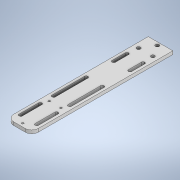
# Autodesk Inventor part: Adapter_Handgelenk_HallsensorHalter
Saved by Autodesk Inventor 2022.2 (Build 262287010, 287A)
## iProperties
Created: 2024-02-12
Part Number: Adapter_Handgelenk_HallsensorHalter
Material: Generisch
Document SubType Name: Modeling
Designer: ppovolni
Density: 1 g/cm^3
Appearance: Vorgabe
Author: ppovolni
Autodesk Inventor part; units mm, degrees
ref_plane "Arbeitsebene1" through (19.8074, 22.7962, -37.1968) normal (0, 1, 0) x (-1, 0, 0)
sketch "Skizze1" plane through (19.8074, 22.7962, -37.1968) normal (0, 1, 0) x (-1, 0, 0)
  circle A0 centre (8, 25) radius 2.8 projected
  circle A1 centre (30, 25) radius 2.8 projected
  circle A2 centre (19, 7) radius 2.8 projected
  spline S0 degree 3 poles (1.3145, 2) (1.0175, 2) (0.7205, 1.9713) (0.2844, 1.885) (0.1411, 1.8492) (0, 1.8064) knots 2.611891 2.611891 2.611891 2.611891 2.701 2.701 2.745234 2.745234 2.745234 2.745234 projected
  line L0 (36.6855, 2) -> (1.3145, 2) projected
  spline S1 degree 3 poles (38, 1.8064) (37.5746, 1.9355) (37.13, 2) (36.6855, 2) knots 0.725365 0.725365 0.725365 0.725365 0.858708 0.858708 0.858708 0.858708 projected
  line L1 (38, 1.8064) -> (38, 28) projected
  spline S2 degree 3 poles (35.7631, 30) (36.052, 30) (36.3933, 29.9384) (36.9135, 29.7364) (37.1885, 29.5671) (37.5676, 29.2109) (37.7437, 28.9664) (37.9403, 28.5182) (38, 28.2384) (38, 28) knots 0.951911 0.951911 0.951911 0.951911 1.038602 1.038602 1.119337 1.119337 1.19466 1.19466 1.266177 1.266177 1.266177 1.266177 projected
  line L2 (2.2369, 30) -> (35.7631, 30) projected
  spline S3 degree 3 poles (0, 28) (0, 28.2384) (0.0597, 28.5182) (0.2563, 28.9664) (0.4324, 29.2109) (0.8115, 29.5671) (1.0865, 29.7364) (1.6067, 29.9384) (1.948, 30) (2.2369, 30) knots 1.266177 1.266177 1.266177 1.266177 1.337694 1.337694 1.413017 1.413017 1.493752 1.493752 1.580443 1.580443 1.580443 1.580443 projected
  line L3 (0, 1.8064) -> (0, 28) projected
  point P0 (19.8074, 37.1968)
ref_plane "Arbeitsebene2" through (19.8074, 22.7962, -37.1968) normal (0, 1, 0) x (-1, 0, 0)
sketch "Skizze2" plane through (19.8074, 22.7962, -37.1968) normal (0, 1, 0) x (-1, 0, 0)
  line L0 (38, 220) -> (0, 220)
  line L1 (0, 220) -> (0, 2)
  line L2 (0, 2) -> (38, 2)
  line L3 (38, 2) -> (38, 220)
  line L4 (38, 1.8064) -> (38, 28) construction
  line L5 (36.6855, 2) -> (1.3145, 2) construction
  line L6 (0, 1.8064) -> (0, 28) construction
  circle A0 centre (8, 25) radius 2.8 construction
  circle A1 centre (19, 7) radius 2.8 construction
  circle A2 centre (19, 7) radius 2.8 construction
  circle A3 centre (30, 25) radius 2.8 construction
  line L7 (24, 205) -> (14, 205) construction
  line L8 (14, 205) -> (14, 185) construction
  line L9 (14, 185) -> (24, 185) construction
  line L10 (24, 185) -> (24, 205) construction
  circle A4 centre (24, 205) radius 1 construction
  circle A5 centre (14, 205) radius 1 construction
  circle A6 centre (24, 185) radius 1 construction
  circle A7 centre (14, 185) radius 1 construction
  line L11 (28, 215) -> (10, 215) construction
  line L12 (10, 215) -> (10, 165) construction
  line L13 (10, 165) -> (28, 165) construction
  line L14 (28, 165) -> (28, 215) construction
  circle A8 centre (28, 165) radius 1.55
  circle A9 centre (10, 165) radius 1.55
  circle A10 centre (19, 215) radius 1.55
  line L15 (5.3985, -5) -> (32.6015, -5) construction
  circle A11 centre (30, 25) radius 2.8 projected
  circle A12 centre (19, 7) radius 2.8 projected
  circle A13 centre (8, 25) radius 2.8 projected
  point P0 (19.8074, 37.1968)
  point P1 (19, 205)
  point P2 (19, 220)
  dimension "d0" = 10
  dimension "d1" = 20
  dimension "d2" = 2
  dimension "d3" = 10
  dimension "d4" = 18
  dimension "d5" = 50
  dimension "d6" = 3.1
  dimension "d8" = 220
  dimension "d9" = 5
  constraints: 24 end point, 7 centre point, 7 coincident, 6 parallel, 5 equal radius, 3 collinear, 3 horizontal, 3 midpoint, 3 perpendicular, 2 vertical alignment
  measures "d0" distance of L7.start L7.end
  measures "d1" distance of L9.end L7.start
  measures "d2" diameter of A5
  measures "d3" distance between parallel lines of L11 L7
  measures "d4" distance of L11.start L11.end
  measures "d5" distance of L13.end L11.start
  measures "d6" diameter of A8
  measures "d8" distance between parallel lines of L11 L15
  measures "d9" distance between parallel lines of L0 L11
extrude "Extrusion1" add sketch "Skizze2" along normal blind 5
sketch "Skizze3" plane through (19.8074, 22.7962, -37.1968) normal (0, -1, 0) x (1, 0, 0)
  line L0 (-15, 30) -> (-23, 30)
  line L1 (-23, 30) -> (-23, 210)
  line L2 (-23, 210) -> (-15, 210)
  line L3 (-15, 210) -> (-15, 30)
  line L4 (-38, 220) -> (0, 220) construction
  line L5 (-29.247, 30) -> (-8.753, 30) construction
  point P0 (-19.8074, 37.1968)
  point P1 (-19, 210)
  point P2 (-19, 220)
  point P3 (-19, 30)
  dimension "d12" = 0
  dimension "d13" = 8
  dimension "d14" = 10
  constraints: 8 end point, 3 midpoint, 2 parallel, 1 horizontal, 1 perpendicular, 1 vertical alignment
  measures "d12" distance from line of point (-19, 30) L5
  measures "d13" distance between parallel lines of L1 L3
  measures "d14" distance from line of L4 point (-19, 210)
ref_plane "Arbeitsebene3" through (-12.7983, 15.7405, -42.1968) normal (0, -1, 0) x (1, 0, 0)
extrude "Extrusion2" add sketch "Skizze3" along normal blind 10
fillet "Rundung1" radius 2 3 edges at (-3.1926, 22.7962, 82.8032) (0.8074, 22.7962, 172.8032) (4.8074, 22.7962, 82.8032)
fillet "Rundung2" radius 10 2 edges at (-18.1926, 25.2962, 182.8032) (19.8074, 25.2962, 182.8032)
fillet "Rundung3" radius 2 4 edges at (-3.1926, 12.7962, 82.8032) (0.8074, 12.7962, 172.8032) (4.8074, 12.7962, 82.8032) (0.8074, 12.7962, -7.1968)
sketch "Skizze4" plane through (19.8074, 22.7962, -37.1968) normal (0, 1, 0) x (1, 0, 0)
  line L0 (-28, -102) -> (-28, -62) construction
  line L1 (-38, -2) -> (-38, -220) construction
  line L2 (0, -2) -> (-38, -2) construction
  line L3 (-28, -71.0877) -> (-28, -66.6042)
  line L4 (-28, -66.6042) -> (-28.9936, -66.6042)
  spline S0 degree 2 poles (-28.9936, -66.6042) (-29.4484, -67.1727) (-30.2492, -68.0822) (-30.61, -68.4233) knots 0 0 0 1 2 2 2
  spline S1 degree 2 poles (-30.61, -68.4233) (-31.0797, -68.8731) (-31.7964, -69.2735) (-32.1721, -69.2735) knots 0 0 0 1 2 2 2
  spline S2 degree 2 poles (-32.1721, -69.2735) (-32.5972, -69.2735) (-33.052, -68.7644) (-33.052, -68.3096) knots 0 0 0 1 2 2 2
  spline S3 degree 2 poles (-33.052, -68.3096) (-33.052, -68.0773) (-32.9383, -67.662) (-32.8494, -67.4495) knots 0 0 0 1 2 2 2
  spline S4 degree 2 poles (-32.8494, -67.4495) (-32.7554, -67.2419) (-32.5577, -66.9453) (-32.5083, -66.8711) knots 0 0 0 1 2 2 2
  line L5 (-32.5083, -66.8711) -> (-32.5083, -66.7525)
  line L6 (-32.5083, -66.7525) -> (-33.838, -66.7525)
  spline S5 degree 2 poles (-33.838, -66.7525) (-33.9616, -67.0095) (-34.2186, -68.1069) (-34.2186, -68.6161) knots 0 0 0 1 2 2 2
  spline S6 degree 2 poles (-34.2186, -68.6161) (-34.2186, -69.7036) (-33.2498, -70.8208) (-32.3748, -70.8208) knots 0 0 0 1 2 2 2
  spline S7 degree 2 poles (-32.3748, -70.8208) (-31.836, -70.8208) (-30.7979, -70.3116) (-30.2047, -69.7234) knots 0 0 0 1 2 2 2
  spline S8 degree 2 poles (-30.2047, -69.7234) (-29.8389, -69.3526) (-29.2704, -68.6556) (-29.1518, -68.5024) knots 0 0 0 1 2 2 2
  line L7 (-29.1518, -68.5024) -> (-29.1518, -71.0877)
  line L8 (-29.1518, -71.0877) -> (-28, -71.0877)
  line L9 (-28, -76.4314) -> (-28, -71.9479)
  line L10 (-28, -71.9479) -> (-28.9936, -71.9479)
  spline S9 degree 2 poles (-28.9936, -71.9479) (-29.4484, -72.5163) (-30.2492, -73.4259) (-30.61, -73.767) knots 0 0 0 1 2 2 2
  spline S10 degree 2 poles (-30.61, -73.767) (-31.0797, -74.2168) (-31.7964, -74.6172) (-32.1721, -74.6172) knots 0 0 0 1 2 2 2
  spline S11 degree 2 poles (-32.1721, -74.6172) (-32.5972, -74.6172) (-33.052, -74.1081) (-33.052, -73.6533) knots 0 0 0 1 2 2 2
  spline S12 degree 2 poles (-33.052, -73.6533) (-33.052, -73.4209) (-32.9383, -73.0057) (-32.8494, -72.7932) knots 0 0 0 1 2 2 2
  spline S13 degree 2 poles (-32.8494, -72.7932) (-32.7554, -72.5855) (-32.5577, -72.2889) (-32.5083, -72.2148) knots 0 0 0 1 2 2 2
  line L11 (-32.5083, -72.2148) -> (-32.5083, -72.0962)
  line L12 (-32.5083, -72.0962) -> (-33.838, -72.0962)
  spline S14 degree 2 poles (-33.838, -72.0962) (-33.9616, -72.3532) (-34.2186, -73.4506) (-34.2186, -73.9598) knots 0 0 0 1 2 2 2
  spline S15 degree 2 poles (-34.2186, -73.9598) (-34.2186, -75.0473) (-33.2498, -76.1645) (-32.3748, -76.1645) knots 0 0 0 1 2 2 2
  spline S16 degree 2 poles (-32.3748, -76.1645) (-31.836, -76.1645) (-30.7979, -75.6553) (-30.2047, -75.0671) knots 0 0 0 1 2 2 2
  spline S17 degree 2 poles (-30.2047, -75.0671) (-29.8389, -74.6963) (-29.2704, -73.9993) (-29.1518, -73.8461) knots 0 0 0 1 2 2 2
  line L13 (-29.1518, -73.8461) -> (-29.1518, -76.4314)
  line L14 (-29.1518, -76.4314) -> (-28, -76.4314)
  spline S18 degree 2 poles (-31.05, -81.696) (-30.2591, -81.696) (-29.0727, -81.4439) (-28.6723, -81.1621) knots 0 0 0 1 2 2 2
  spline S19 degree 2 poles (-28.6723, -81.1621) (-28.2768, -80.8853) (-27.8715, -79.9906) (-27.8715, -79.3479) knots 0 0 0 1 2 2 2
  spline S20 degree 2 poles (-27.8715, -79.3479) (-27.8715, -78.7004) (-28.2768, -77.8106) (-28.6822, -77.5288) knots 0 0 0 1 2 2 2
  spline S21 degree 2 poles (-28.6822, -77.5288) (-29.0826, -77.247) (-30.2591, -76.9949) (-31.05, -76.9949) knots 0 0 0 1 2 2 2
  spline S22 degree 2 poles (-31.05, -76.9949) (-31.8607, -76.9949) (-33.0075, -77.247) (-33.4228, -77.5338) knots 0 0 0 1 2 2 2
  spline S23 degree 2 poles (-33.4228, -77.5338) (-33.8281, -77.8205) (-34.2236, -78.7251) (-34.2236, -79.3479) knots 0 0 0 1 2 2 2
  spline S24 degree 2 poles (-34.2236, -79.3479) (-34.2236, -80.0054) (-33.8083, -80.8853) (-33.3981, -81.1671) knots 0 0 0 1 2 2 2
  spline S25 degree 2 poles (-33.3981, -81.1671) (-32.9977, -81.4439) (-31.8162, -81.696) (-31.05, -81.696) knots 0 0 0 1 2 2 2
  spline S26 degree 2 poles (-31.05, -80.1586) (-32.182, -80.1586) (-33.0965, -79.7879) (-33.0965, -79.3479) knots 0 0 0 1 2 2 2
  spline S27 degree 2 poles (-33.0965, -79.3479) (-33.0965, -78.908) (-32.182, -78.5323) (-31.0451, -78.5323) knots 0 0 0 1 2 2 2
  spline S28 degree 2 poles (-31.0451, -78.5323) (-29.9279, -78.5323) (-28.9985, -78.908) (-28.9985, -79.3479) knots 0 0 0 1 2 2 2
  spline S29 degree 2 poles (-28.9985, -79.3479) (-28.9985, -79.7829) (-29.9279, -80.1586) (-31.05, -80.1586) knots 0 0 0 1 2 2 2
  line L15 (-28, -88.058) -> (-30.2986, -88.058)
  spline S30 degree 2 poles (-30.2986, -88.058) (-30.6397, -88.058) (-31.1044, -88.0333) (-31.2527, -87.9739) knots 0 0 0 1 2 2 2
  spline S31 degree 2 poles (-31.2527, -87.9739) (-31.401, -87.9097) (-31.5344, -87.6526) (-31.5344, -87.4203) knots 0 0 0 1 2 2 2
  spline S32 degree 2 poles (-31.5344, -87.4203) (-31.5344, -87.2572) (-31.3911, -86.9408) (-31.2576, -86.753) knots 0 0 0 1 2 2 2
  line L16 (-31.2576, -86.753) -> (-28, -86.753)
  line L17 (-28, -86.753) -> (-28, -85.3095)
  line L18 (-28, -85.3095) -> (-30.2986, -85.3095)
  spline S33 degree 2 poles (-30.2986, -85.3095) (-30.6348, -85.3095) (-31.1044, -85.2799) (-31.2527, -85.2205) knots 0 0 0 1 2 2 2
  spline S34 degree 2 poles (-31.2527, -85.2205) (-31.401, -85.1563) (-31.5344, -84.8992) (-31.5344, -84.6669) knots 0 0 0 1 2 2 2
  spline S35 degree 2 poles (-31.5344, -84.6669) (-31.5344, -84.4939) (-31.3713, -84.1528) (-31.2576, -83.9946) knots 0 0 0 1 2 2 2
  line L19 (-31.2576, -83.9946) -> (-28, -83.9946)
  line L20 (-28, -83.9946) -> (-28, -82.5611)
  line L21 (-28, -82.5611) -> (-32.6022, -82.5611)
  line L22 (-32.6022, -82.5611) -> (-32.6022, -83.9946)
  line L23 (-32.6022, -83.9946) -> (-32.093, -83.9946)
  spline S36 degree 2 poles (-32.093, -83.9946) (-32.3896, -84.3456) (-32.7258, -84.9734) (-32.7258, -85.3639) knots 0 0 0 1 2 2 2
  spline S37 degree 2 poles (-32.7258, -85.3639) (-32.7258, -85.7841) (-32.3254, -86.4267) (-31.925, -86.5948) knots 0 0 0 1 2 2 2
  spline S38 degree 2 poles (-31.925, -86.5948) (-32.3105, -87.0051) (-32.7258, -87.7367) (-32.7258, -88.1124) knots 0 0 0 1 2 2 2
  spline S39 degree 2 poles (-32.7258, -88.1124) (-32.7258, -88.4337) (-32.5231, -88.9428) (-32.3155, -89.1158) knots 0 0 0 1 2 2 2
  spline S40 degree 2 poles (-32.3155, -89.1158) (-32.093, -89.3086) (-31.485, -89.5014) (-30.9956, -89.5014) knots 0 0 0 1 2 2 2
  line L24 (-30.9956, -89.5014) -> (-28, -89.5014)
  line L25 (-28, -89.5014) -> (-28, -88.058)
  line L26 (-28, -96.0562) -> (-30.2986, -96.0562)
  spline S41 degree 2 poles (-30.2986, -96.0562) (-30.6397, -96.0562) (-31.1044, -96.0315) (-31.2527, -95.9722) knots 0 0 0 1 2 2 2
  spline S42 degree 2 poles (-31.2527, -95.9722) (-31.401, -95.9079) (-31.5344, -95.6509) (-31.5344, -95.4185) knots 0 0 0 1 2 2 2
  spline S43 degree 2 poles (-31.5344, -95.4185) (-31.5344, -95.2554) (-31.3911, -94.939) (-31.2576, -94.7512) knots 0 0 0 1 2 2 2
  line L27 (-31.2576, -94.7512) -> (-28, -94.7512)
  line L28 (-28, -94.7512) -> (-28, -93.3077)
  line L29 (-28, -93.3077) -> (-30.2986, -93.3077)
  spline S44 degree 2 poles (-30.2986, -93.3077) (-30.6348, -93.3077) (-31.1044, -93.2781) (-31.2527, -93.2188) knots 0 0 0 1 2 2 2
  spline S45 degree 2 poles (-31.2527, -93.2188) (-31.401, -93.1545) (-31.5344, -92.8974) (-31.5344, -92.6651) knots 0 0 0 1 2 2 2
  spline S46 degree 2 poles (-31.5344, -92.6651) (-31.5344, -92.4921) (-31.3713, -92.151) (-31.2576, -91.9928) knots 0 0 0 1 2 2 2
  line L30 (-31.2576, -91.9928) -> (-28, -91.9928)
  line L31 (-28, -91.9928) -> (-28, -90.5593)
  line L32 (-28, -90.5593) -> (-32.6022, -90.5593)
  line L33 (-32.6022, -90.5593) -> (-32.6022, -91.9928)
  line L34 (-32.6022, -91.9928) -> (-32.093, -91.9928)
  spline S47 degree 2 poles (-32.093, -91.9928) (-32.3896, -92.3438) (-32.7258, -92.9716) (-32.7258, -93.3621) knots 0 0 0 1 2 2 2
  spline S48 degree 2 poles (-32.7258, -93.3621) (-32.7258, -93.7823) (-32.3254, -94.4249) (-31.925, -94.593) knots 0 0 0 1 2 2 2
  spline S49 degree 2 poles (-31.925, -94.593) (-32.3105, -95.0033) (-32.7258, -95.7349) (-32.7258, -96.1106) knots 0 0 0 1 2 2 2
  spline S50 degree 2 poles (-32.7258, -96.1106) (-32.7258, -96.4319) (-32.5231, -96.941) (-32.3155, -97.1141) knots 0 0 0 1 2 2 2
  spline S51 degree 2 poles (-32.3155, -97.1141) (-32.093, -97.3068) (-31.485, -97.4996) (-30.9956, -97.4996) knots 0 0 0 1 2 2 2
  line L35 (-30.9956, -97.4996) -> (-28, -97.4996)
  line L36 (-28, -97.4996) -> (-28, -96.0562)
  point P0 (-19.8074, -37.1968)
  point P1 (-38, -210)
  dimension "d20" = 10
  dimension "d21" = 40
  dimension "d22" = 60
  constraints: 2 end point, 2 vertical
  measures "d20" distance between parallel lines of L0 L1
  measures "d21" distance of L0.start L0.end
  measures "d22" distance from line of L2 L0.end
extrude "Extrusion3" add sketch "Skizze4" against normal blind 0.2
sketch "Skizze5" plane through (19.8074, 22.7962, -37.1968) normal (0, -1, 0) x (1, 0, 0)
  line L0 (-6, 157) -> (-7, 157)
  line L1 (-9, 155) -> (-9, 104)
  line L2 (-7, 102) -> (-6, 102)
  line L3 (-4, 104) -> (-4, 155)
  line L4 (-6, 64) -> (-7, 64)
  line L5 (-9, 62) -> (-9, 41)
  line L6 (-7, 39) -> (-6, 39)
  line L7 (-4, 41) -> (-4, 62)
  line L8 (-31, 157) -> (-32, 157)
  line L9 (-34, 155) -> (-34, 104)
  line L10 (-32, 102) -> (-31, 102)
  line L11 (-29, 104) -> (-29, 155)
  line L12 (-31, 64) -> (-32, 64)
  line L13 (-34, 62) -> (-34, 41)
  line L14 (-32, 39) -> (-31, 39)
  line L15 (-29, 41) -> (-29, 62)
  line L16 (-6, 208) -> (-7, 208)
  line L17 (-9, 206) -> (-9, 175)
  line L18 (-7, 173) -> (-6, 173)
  line L19 (-4, 175) -> (-4, 206)
  line L20 (-31, 208) -> (-32, 208)
  line L21 (-34, 206) -> (-34, 175)
  line L22 (-32, 173) -> (-31, 173)
  line L23 (-29, 175) -> (-29, 206)
  line L24 (-13, 30) -> (-13, 212) projected
  line L25 (0, 210) -> (0, 2) projected
  line L26 (-38, 2) -> (-38, 210) projected
  line L27 (-28, 220) -> (-10, 220) projected
  arc A0 (-4, 206) -> (-6, 208) centre (-6, 206) ccw
  arc A1 (-7, 208) -> (-9, 206) centre (-7, 206) ccw
  arc A2 (-6, 173) -> (-4, 175) centre (-6, 175) ccw
  arc A3 (-9, 175) -> (-7, 173) centre (-7, 175) ccw
  arc A4 (-31, 173) -> (-29, 175) centre (-31, 175) ccw
  arc A5 (-34, 175) -> (-32, 173) centre (-32, 175) ccw
  arc A6 (-29, 206) -> (-31, 208) centre (-31, 206) ccw
  arc A7 (-32, 208) -> (-34, 206) centre (-32, 206) ccw
  arc A8 (-29, 155) -> (-31, 157) centre (-31, 155) ccw
  arc A9 (-32, 157) -> (-34, 155) centre (-32, 155) ccw
  arc A10 (-4, 155) -> (-6, 157) centre (-6, 155) ccw
  arc A11 (-7, 157) -> (-9, 155) centre (-7, 155) ccw
  arc A12 (-6, 102) -> (-4, 104) centre (-6, 104) ccw
  arc A13 (-9, 104) -> (-7, 102) centre (-7, 104) ccw
  arc A14 (-31, 102) -> (-29, 104) centre (-31, 104) ccw
  arc A15 (-34, 104) -> (-32, 102) centre (-32, 104) ccw
  arc A16 (-4, 62) -> (-6, 64) centre (-6, 62) ccw
  arc A17 (-7, 64) -> (-9, 62) centre (-7, 62) ccw
  arc A18 (-6, 39) -> (-4, 41) centre (-6, 41) ccw
  arc A19 (-9, 41) -> (-7, 39) centre (-7, 41) ccw
  arc A20 (-31, 39) -> (-29, 41) centre (-31, 41) ccw
  arc A21 (-34, 41) -> (-32, 39) centre (-32, 41) ccw
  arc A22 (-29, 62) -> (-31, 64) centre (-31, 62) ccw
  arc A23 (-32, 64) -> (-34, 62) centre (-32, 62) ccw
  point P0 (-19.8074, 37.1968)
  point P1 (-4, 157)
  point P2 (-4, 102)
  point P3 (-4, 64)
  point P4 (-29, 64)
  point P5 (-34, 39)
  point P6 (-34, 64)
  point P7 (-4, 208)
  point P8 (-9, 173)
  point P9 (-4, 173)
  point P10 (-34, 173)
  point P11 (-6.5, 208)
  point P12 (-6.5, 173)
  point P13 (-31.5, 102)
  dimension "d25" = 5
  dimension "d26" = 5
  dimension "d27" = 13
  dimension "d28" = 4
  dimension "d29" = 4
  dimension "d30" = 12
  dimension "d31" = 35
  dimension "d32" = 16
  dimension "d33" = 55
  dimension "d34" = 38
  dimension "d35" = 25
  dimension "d36" = 2
  dimension "d37" = 2
  constraints: 48 end point, 48 point on circle, 48 tangent, 26 point on line, 24 centre point, 22 equal radius, 12 parallel, 8 collinear, 6 horizontal, 6 perpendicular, 3 midpoint
  measures "d25" distance between parallel lines of L17 L19
  measures "d26" distance between parallel lines of L21 L23
  measures "d27" distance between parallel lines of L24 L25
  measures "d28" distance between parallel lines of L19 L25
  measures "d29" distance between parallel lines of L26 L21
  measures "d30" distance from line of L27 point (-6.5, 208)
  measures "d31" distance of point (-4, 173) point (-4, 208)
  measures "d32" distance from line of L0 point (-6.5, 173)
  measures "d33" distance of point (-4, 102) point (-4, 157)
  measures "d34" distance from line of point (-31.5, 102) L12
  measures "d35" distance of point (-34, 64) point (-34, 39)
  measures "d36" radius of A0
  measures "d37" radius of A12
extrude "Extrusion4" cut sketch "Skizze5" against normal through all
